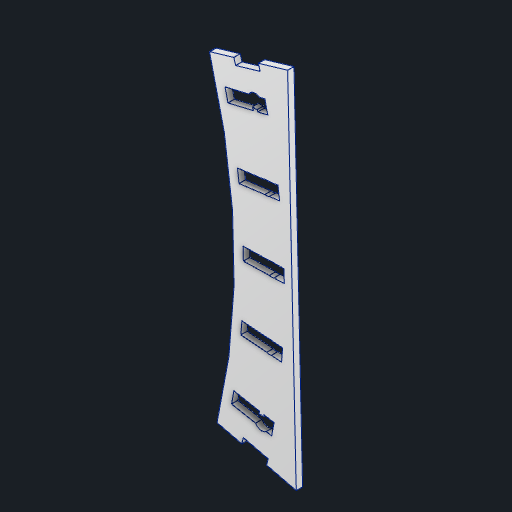
# Autodesk Inventor part: Back Plate
Saved by Autodesk Inventor 2023 (Build 270158000, 158)
## iProperties
Created: 2022-06-13
Part Number: Back Plate
Material: Aluminum 6061
Document SubType Name: Modeling
Designer: FizzyApple12
Density: 2.7 g/cm^3
Appearance: Aluminum - Flat
Author: FizzyApple12
Autodesk Inventor part; units mm, degrees
ref_plane "YZ Plane" through (0, 0, 0) normal (1, 0, 0) x (0, 1, 0)
ref_plane "XZ Plane" through (0, 0, 0) normal (0, 1, 0) x (-1, 0, 0)
ref_plane "Work Plane2" through (388.0538, -686.9281, 216.8066) normal (0, 0, 1) x (-0.9917, -0.1283, 0)
sketch "Sketch3" plane through (388.0538, -686.9281, 216.8066) normal (0, 0, 1) x (-0.9917, -0.1283, 0)
  line L0 (4.3583, 15.8159) -> (10.8533, 46.3726) construction
  line L1 (1.0044, -15.8113) -> (4.2698, 15.2569) construction
  line L2 (1.0044, -15.8113) -> (4.2698, 15.2569) construction
  line L3 (0.9748, -47.6157) -> (0.9748, -16.3764) construction
  line L4 (0.9748, -47.6157) -> (0.9748, -16.3764) construction
  line L5 (4.2698, -79.2491) -> (1.0044, -48.1809) construction
  line L6 (4.2698, -79.2491) -> (1.0044, -48.1809) construction
  line L7 (10.9998, 46.9192) -> (20.6533, 76.6296) construction
  line L8 (4.3583, 15.8159) -> (10.8533, 46.3726) construction
  line L9 (10.9998, 46.9192) -> (20.6533, 76.6296) construction
  line L10 (20.6533, 76.6296) -> (-103.8397, 124.4179) construction
  line L11 (-117.8064, 81.4327) -> (10.9998, 46.9192) construction
  line L12 (10.8533, 46.3726) -> (-117.9529, 80.8861) construction
  line L13 (-127.3499, 36.6764) -> (4.3583, 15.8159) construction
  line L14 (4.2698, 15.2569) -> (-127.4385, 36.1175) construction
  line L15 (0.9748, -16.3764) -> (-132.1925, -9.3974) construction
  line L16 (-132.1629, -8.8323) -> (1.0044, -15.8113) construction
  line L17 (1.0044, -48.1809) -> (-132.1629, -55.1599) construction
  line L18 (-132.1925, -54.5947) -> (0.9748, -47.6157) construction
  line L19 (-127.4385, -100.1096) -> (4.2698, -79.2491) construction
  line L20 (19.0965, 77.2271) -> (9.3891, 47.3508)
  line L21 (9.3891, 47.3508) -> (9.2426, 46.8041)
  line L22 (9.2426, 46.8041) -> (2.7113, 16.0767)
  line L23 (2.7113, 16.0767) -> (2.6228, 15.5178)
  line L24 (2.6228, 15.5178) -> (-0.6609, -15.724)
  line L25 (-0.6609, -15.724) -> (-0.6905, -16.2891)
  line L26 (-0.6905, -16.2891) -> (-0.6905, -47.703)
  line L27 (-0.6905, -47.703) -> (-0.6609, -48.2681)
  line L28 (-0.6609, -48.2681) -> (2.6228, -79.5099)
  line L29 (2.6228, -79.5099) -> (-36.3059, -75.4184)
  line L30 (-36.3059, -75.4184) -> (-19.8322, 81.3187)
  line L31 (-19.8322, 81.3187) -> (19.0965, 77.2271)
  line L32 (-127.4385, 36.1175) -> (-129.1369, 19.9578) construction
  point P0 (296.7492, -731.0239)
  dimension "d32" = 1.6652
  dimension "d33" = 1.6652
  dimension "d34" = 1.6652
  dimension "d35" = 1.6652
  dimension "d36" = 1.6652
  dimension "d37" = 29.21
  constraints: 24 end point, 10 point on line, 8 parallel, 1 perpendicular
  measures "d32" distance between parallel lines of L1 L24
  measures "d33" distance between parallel lines of L22 L0
  measures "d34" distance between parallel lines of L20 L7
  measures "d35" distance between parallel lines of L26 L3
  measures "d36" distance between parallel lines of L6 L28
  measures "d37" distance between parallel lines of L30 L24
extrude "Extrusion3" add sketch "Sketch3" along normal blind 3.175
sketch "Sketch5" plane through (388.0538, -686.9281, 219.9816) normal (0, 0, 1) x (0.9917, 0.1283, 0)
  line L0 (-19.0965, -77.2271) -> (19.8322, -81.3187) projected
  line L1 (-19.0965, -77.2271) -> (-19.1979, -77.4913)
  line L2 (-19.1979, -77.4913) -> (-7.3415, -82.0426)
  line L3 (4.515, -86.5938) -> (18.7052, -92.0409)
  line L4 (19.8322, -81.3187) -> (36.3059, 75.4184) projected
  line L5 (19.8322, -81.3187) -> (18.7052, -92.0409)
  line L6 (-18.0601, -74.5272) -> (-19.1979, -77.4913) construction
  line L7 (36.3059, 75.4184) -> (37.4328, 86.1406)
  line L8 (37.4328, 86.1406) -> (22.4202, 83.7628)
  line L9 (9.8766, 81.7761) -> (-2.6671, 79.7894)
  line L10 (36.3059, 75.4184) -> (-2.6228, 79.5099) projected
  line L11 (-2.6671, 79.7894) -> (-2.6228, 79.5099)
  line L12 (-2.6671, 79.7894) -> (-2.1704, 76.6535) construction
  line L13 (1.5509, -85.456) -> (-4.3773, -83.1804) projected
  line L14 (2.6887, -82.4919) -> (1.5509, -85.456) projected
  line L15 (-3.2395, -80.2163) -> (2.6887, -82.4919) projected
  line L16 (-3.2395, -80.2163) -> (-4.3773, -83.1804) projected
  line L17 (19.781, 80.1302) -> (13.5092, 79.1369) projected
  line L18 (19.2843, 83.2662) -> (19.781, 80.1302) projected
  line L19 (13.0125, 82.2728) -> (19.2843, 83.2662) projected
  line L20 (13.0125, 82.2728) -> (13.5092, 79.1369) projected
  line L21 (-4.3773, -83.1804) -> (-7.3415, -82.0426) projected
  line L22 (-3.2395, -80.2163) -> (-4.3773, -83.1804) projected
  line L23 (-6.2036, -79.0785) -> (-3.2395, -80.2163) projected
  line L24 (-7.3415, -82.0426) -> (-6.2036, -79.0785) projected
  line L25 (4.515, -86.5938) -> (1.5509, -85.456) projected
  line L26 (5.6528, -83.6297) -> (4.515, -86.5938) projected
  line L27 (2.6887, -82.4919) -> (5.6528, -83.6297) projected
  line L28 (2.6887, -82.4919) -> (1.5509, -85.456) projected
  line L29 (22.9169, 80.6269) -> (19.781, 80.1302) projected
  line L30 (22.4202, 83.7628) -> (22.9169, 80.6269) projected
  line L31 (19.2843, 83.2662) -> (22.4202, 83.7628) projected
  line L32 (19.2843, 83.2662) -> (19.781, 80.1302) projected
  line L33 (13.5092, 79.1369) -> (10.3733, 78.6402) projected
  line L34 (13.0125, 82.2728) -> (13.5092, 79.1369) projected
  line L35 (9.8766, 81.7761) -> (13.0125, 82.2728) projected
  line L36 (10.3733, 78.6402) -> (9.8766, 81.7761) projected
  point P0 (-296.7492, 731.0239)
  point P1 (19.781, 80.1302)
  point P2 (13.5092, 79.1369)
  point P3 (2.6887, -82.4919)
  constraints: 16 end point, 4 collinear, 3 parallel, 1 perpendicular
extrude "Extrusion4" add sketch "Sketch5" against normal blind 3.175 contours L10 L11 L9 L36 L33 L17 L29 L30 L8 L7 | L0 L5 L3 L26 L27 L15 L23 L24 L2 L1
sketch "Sketch6" plane through (388.0538, -686.9281, 219.9816) normal (0, 0, 1) x (0.9917, 0.1283, 0)
  line L0 (16.6451, 79.6336) -> (18.6318, 67.0899) construction
  line L1 (-0.2754, -81.3541) -> (4.2759, -69.4976) construction
  line L2 (18.7052, -92.0409) -> (37.4328, 86.1406) construction
  line L3 (28.069, -2.9502) -> (17.9647, -1.8882) construction
  line L4 (-6.2036, -79.0785) -> (5.6528, -83.6297) construction
  line L5 (22.9169, 80.6269) -> (10.3733, 78.6402) construction
  point P0 (-296.7492, 731.0239)
  dimension "d23" = 12.7
  dimension "d24" = 12.7
  dimension "d55" = 10.16
  constraints: 6 end point, 3 coincident, 3 midpoint, 3 perpendicular
  measures "d23" distance of L0.start L0.end
  measures "d24" distance of L1.start L1.end
  measures "d55" distance from line of L3.end L2
hole "Hole2" at (401.2076, -755.3034, 219.9816) at (397.9274, -618.0027, 219.9816) at (406.1123, -686.4967, 219.9816) direction (0, 0, -1) diameter 6.7564 depth 13.6144 clearance for "Flat Head Machine Screw (82)" size "1/4" standard "Ansi Unified Screw Threads"
sketch "Sketch7" plane through (388.0538, -686.9281, 219.9816) normal (0, 0, 1) x (0.9917, 0.1283, 0)
  line L0 (0.6609, 15.724) -> (-2.6228, -15.5178) construction
  line L1 (-0.981, 0.1031) -> (10.3864, -1.0917) construction
  line L2 (3.6239, -3.5734) -> (16.4852, -4.9251)
  line L3 (16.4852, -4.9251) -> (17.1489, 1.3901)
  line L4 (17.1489, 1.3901) -> (4.2877, 2.7418)
  line L5 (4.2877, 2.7418) -> (3.6239, -3.5734)
  line L6 (3.6239, -3.5734) -> (17.1489, 1.3901) construction
  line L7 (16.4852, -4.9251) -> (4.2877, 2.7418) construction
  circle A0 centre (17.9647, -1.8882) radius 3.3782 construction
  line L8 (10.8679, -38.2669) -> (-1.7816, -35.5781)
  line L9 (-1.7816, -35.5781) -> (-0.4614, -29.3669)
  line L10 (-0.4614, -29.3669) -> (12.1881, -32.0556)
  line L11 (12.1881, -32.0556) -> (10.8679, -38.2669)
  line L12 (10.8679, -38.2669) -> (-0.4614, -29.3669) construction
  line L13 (-1.7816, -35.5781) -> (12.1881, -32.0556) construction
  line L14 (-10.5029, -66.8425) -> (1.7962, -70.8387)
  line L15 (1.7962, -70.8387) -> (3.7585, -64.7995)
  line L16 (3.7585, -64.7995) -> (-8.5407, -60.8033)
  line L17 (-8.5407, -60.8033) -> (-10.5029, -66.8425)
  line L18 (-10.5029, -66.8425) -> (3.7585, -64.7995) construction
  line L19 (1.7962, -70.8387) -> (-8.5407, -60.8033) construction
  line L20 (18.5865, 35.1711) -> (5.6544, 35.1711)
  line L21 (5.6544, 35.1711) -> (5.6544, 28.8211)
  line L22 (5.6544, 28.8211) -> (18.5865, 28.8211)
  line L23 (18.5865, 28.8211) -> (18.5865, 35.1711)
  line L24 (18.5865, 35.1711) -> (5.6544, 28.8211) construction
  line L25 (5.6544, 35.1711) -> (18.5865, 28.8211) construction
  line L26 (3.6239, 67.5655) -> (4.2877, 61.2503)
  line L27 (4.2877, 61.2503) -> (17.1489, 62.6021)
  line L28 (17.1489, 62.6021) -> (16.4852, 68.9173)
  line L29 (16.4852, 68.9173) -> (3.6239, 67.5655)
  line L30 (3.6239, 67.5655) -> (17.1489, 62.6021) construction
  line L31 (4.2877, 61.2503) -> (16.4852, 68.9173) construction
  line L32 (-9.3891, -47.3508) -> (-19.0965, -77.2271) construction
  line L33 (-14.2428, -62.289) -> (-3.3722, -65.821) construction
  line L34 (-2.7113, -16.0767) -> (-9.2426, -46.8041) construction
  line L35 (-5.977, -31.4404) -> (5.2033, -33.8169) construction
  line L36 (0.6905, 47.703) -> (0.6905, 16.2891) construction
  line L37 (0.6905, 31.9961) -> (12.1205, 31.9961) construction
  line L38 (-2.6228, 79.5099) -> (0.6609, 48.2681) construction
  line L39 (-0.981, 63.889) -> (10.3864, 65.0838) construction
  line L40 (18.7804, -5.1664) -> (19.4442, 1.1488)
  line L41 (19.4442, 1.1488) -> (24.4964, 0.6178)
  line L42 (24.4964, 0.6178) -> (23.8326, -5.6974)
  line L43 (23.8326, -5.6974) -> (18.7804, -5.1664)
  line L44 (18.7804, -5.1664) -> (24.4964, 0.6178) construction
  line L45 (19.4442, 1.1488) -> (23.8326, -5.6974) construction
  line L46 (13.1254, -38.7467) -> (14.4456, -32.5355)
  line L47 (14.4456, -32.5355) -> (19.4146, -33.5916)
  line L48 (19.4146, -33.5916) -> (18.0943, -39.8029)
  line L49 (18.0943, -39.8029) -> (13.1254, -38.7467)
  line L50 (13.1254, -38.7467) -> (19.4146, -33.5916) construction
  line L51 (14.4456, -32.5355) -> (18.0943, -39.8029) construction
  line L52 (20.8944, 28.8211) -> (20.8944, 35.1711)
  line L53 (20.8944, 35.1711) -> (25.9744, 35.1711)
  line L54 (25.9744, 35.1711) -> (25.9744, 28.8211)
  line L55 (25.9744, 28.8211) -> (20.8944, 28.8211)
  line L56 (20.8944, 28.8211) -> (25.9744, 35.1711) construction
  line L57 (20.8944, 35.1711) -> (25.9744, 28.8211) construction
  line L58 (3.9912, -71.5519) -> (5.9534, -65.5127)
  line L59 (5.9534, -65.5127) -> (10.7848, -67.0825)
  line L60 (10.7848, -67.0825) -> (8.8225, -73.1217)
  line L61 (8.8225, -73.1217) -> (3.9912, -71.5519)
  line L62 (3.9912, -71.5519) -> (10.7848, -67.0825) construction
  line L63 (5.9534, -65.5127) -> (8.8225, -73.1217) construction
  line L64 (19.4442, 62.8433) -> (18.7804, 69.1585)
  line L65 (18.7804, 69.1585) -> (23.8326, 69.6895)
  line L66 (23.8326, 69.6895) -> (24.4964, 63.3743)
  line L67 (24.4964, 63.3743) -> (19.4442, 62.8433)
  line L68 (19.4442, 62.8433) -> (23.8326, 69.6895) construction
  line L69 (18.7804, 69.1585) -> (24.4964, 63.3743) construction
  point P0 (-296.7492, 731.0239)
  point P1 (5.2033, -33.8169)
  point P2 (-3.3722, -65.821)
  point P3 (12.1205, 31.9961)
  point P4 (10.3864, 65.0838)
  point P5 (21.6384, -2.2743)
  dimension "d38" = 11.43
  dimension "d39" = 6.35
  dimension "d40" = 12.9321
  dimension "d41" = 11.43
  dimension "d42" = 11.43
  dimension "d43" = 11.43
  dimension "d44" = 11.43
  dimension "d45" = 6.35
  dimension "d46" = 6.35
  dimension "d47" = 6.35
  dimension "d48" = 6.35
  dimension "d49" = 12.9321
  dimension "d50" = 12.9321
  dimension "d51" = 12.9321
  dimension "d52" = 12.9321
  dimension "d66" = 6.35
  dimension "d67" = 5.08
  dimension "d68" = 2.3079
  dimension "d69" = 6.35
  dimension "d70" = 5.08
  dimension "d71" = 6.35
  dimension "d72" = 5.08
  dimension "d73" = 6.35
  dimension "d74" = 5.08
  dimension "d75" = 6.35
  dimension "d76" = 5.08
  dimension "d77" = 2.3079
  dimension "d78" = 2.3079
  dimension "d79" = 2.3079
  dimension "d80" = 2.3079
  constraints: 130 end point, 25 parallel, 21 midpoint, 20 perpendicular, 4 collinear, 3 point on circle
  measures "d38" distance of L1.start L1.end
  measures "d39" distance of L3.end L2.end
  measures "d40" distance between parallel lines of L3 L5
  measures "d41" distance of L33.end L33.start
  measures "d42" distance of L35.end L35.start
  measures "d43" distance of L37.end L37.start
  measures "d44" distance of L39.end L39.start
  measures "d45" distance between parallel lines of L14 L16
  measures "d46" distance between parallel lines of L22 L20
  measures "d47" distance between parallel lines of L8 L10
  measures "d48" distance between parallel lines of L29 L27
  measures "d49" distance between parallel lines of L28 L26
  measures "d50" distance between parallel lines of L21 L23
  measures "d51" distance between parallel lines of L9 L11
  measures "d52" distance between parallel lines of L17 L15
  measures "d66" distance of L40.start L40.end
  measures "d67" distance between parallel lines of L40 L42
  measures "d68" distance between parallel lines of L40 L3
  measures "d69" distance of L50.start L51.start
  measures "d70" distance between parallel lines of L46 L48
  measures "d71" distance of L56.start L57.start
  measures "d72" distance between parallel lines of L52 L54
  measures "d73" distance of L62.start L63.start
  measures "d74" distance between parallel lines of L58 L60
  measures "d75" distance of L68.start L69.start
  measures "d76" distance between parallel lines of L64 L66
  measures "d77" distance between parallel lines of L11 L46
  measures "d78" distance between parallel lines of L15 L58
  measures "d79" distance between parallel lines of L23 L52
  measures "d80" distance between parallel lines of L28 L64
extrude "Extrusion5" cut sketch "Sketch7" against normal blind 3.175
sketch "Sketch8" plane through (388.0538, -686.9281, 219.9816) normal (0, 0, 1) x (0.9917, 0.1283, 0)
  line L0 (0.6609, 15.724) -> (-2.6228, -15.5178) construction
  arc A0 (16.4852, -4.9251) -> (17.1489, 1.3901) centre (17.9647, -1.8882) ccw construction
  line L1 (18.5865, 35.1711) -> (18.5865, 28.8211) construction
  line L2 (18.5865, 31.9961) -> (19.7405, 31.9961) construction
  line L3 (0.6905, 47.703) -> (0.6905, 16.2891) construction
  line L4 (10.8679, -38.2669) -> (12.1881, -32.0556) construction
  line L5 (11.528, -35.1612) -> (12.6567, -35.4012) construction
  line L6 (-2.7113, -16.0767) -> (-9.2426, -46.8041) construction
  point P0 (-296.7492, 731.0239)
  point P1 (-0.6491, 3.2607)
  point P2 (0.6905, 35.1711)
  point P3 (-5.3169, -28.3348)
  dimension "d56" = 19.05
  dimension "d57" = 19.05
  dimension "d58" = 19.05
  constraints: 4 end point, 2 coincident, 2 midpoint, 2 perpendicular
  measures "d56" distance from line of L0 A0.centre
  measures "d57" distance from line of L3 L2.end
  measures "d58" distance from line of L6 point (12.657, -35.401)
hole "Hole3" at (403.5277, -652.6645, 219.9816) at (405.1463, -720.4137, 219.9816) direction (0, 0, -1) diameter 6.7564 depth 13.6144 clearance for "Flat Head Machine Screw (82)" size "1/4" standard "Ansi Unified Screw Threads"
equation "\"d33\" = d32"
equation "\"d34\" = d32"
equation "\"d36\" = d32"
equation "\"d41\" = d38"
equation "\"d42\" = d38"
equation "\"d43\" = d38"
equation "\"d44\" = d38"
equation "\"d45\" = d39"
equation "\"d46\" = d39"
equation "\"d47\" = d39"
equation "\"d48\" = d39"
equation "\"d49\" = d40"
equation "\"d50\" = d40"
equation "\"d51\" = d40"
equation "\"d52\" = d40"
equation "\"d57\" = d56"
equation "\"d58\" = d56"
body "Solid3"
